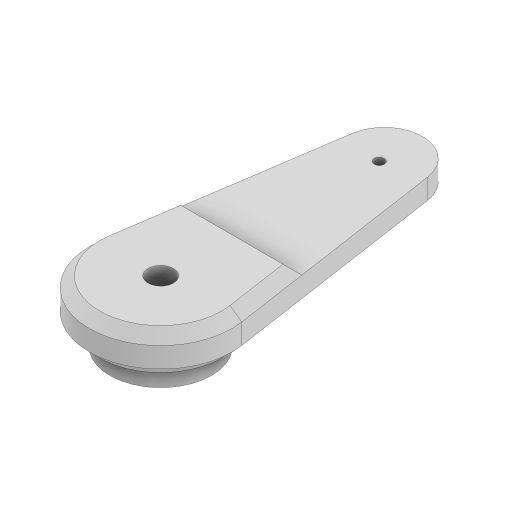
# Autodesk Inventor part: 5P.00.18.01-IB-VTP-Servo-Horn
Saved by Autodesk Inventor 2024.3 (Build 283343000, 343)
## iProperties
Created: 2025-01-15
Part Number: 5P.00.18.01-IB-VTP-Servo-Horn
Material: Generic
Document SubType Name: Modeling
Designer: inigo
Density: 1 g/cm^3
Appearance: Default
Author: inigo
Autodesk Inventor part; units mm, degrees
ref_plane "YZ Plane" through (0, 0, 0) normal (1, 0, 0) x (0, 1, 0)
ref_plane "XZ Plane" through (0, 0, 0) normal (0, 1, 0) x (-1, 0, 0)
sketch "Sketch1" plane through (0, 0, 0) normal (0, 1, 0) x (-1, 0, 0)
  arc A0 (6.9232, -1.0341) -> (-6.9232, -1.0341) centre (0, 0) ccw
  arc A1 (-3.7089, -22.554) -> (3.7089, -22.554) centre (0, -22) ccw
  line L0 (6.9232, -1.0341) -> (3.7089, -22.554)
  line L1 (-6.9232, -1.0341) -> (-3.7089, -22.554)
  circle A2 centre (0, -21.5) radius 0.5
  dimension "d0" = 14
  dimension "d1" = 7.5
  dimension "d2" = 22
  dimension "d3" = 1
  dimension "d4" = 21.5
  constraints: 4 end point, 4 point on circle, 4 tangent, 3 centre point, 2 vertical alignment, 1 coincident
  measures "d0" diameter of A0
  measures "d1" diameter of A1
  measures "d2" distance of A1.centre point (0, 0)
  measures "d3" diameter of A2
  measures "d4" distance of point (0, 0) A2.centre
extrude "Extrusion1" add sketch "Sketch1" along normal blind 2
sketch "Sketch2" plane through (0, 2, 0) normal (0, 1, 0) x (1, 0, 0)
  line L0 (-3.7089, 22.554) -> (-6.9232, 1.0341) projected
  line L1 (-5.8827, 8) -> (5.8827, 8)
  line L2 (6.9232, 1.0341) -> (3.7089, 22.554) projected
  arc A0 (-6.9232, 1.0341) -> (6.9232, 1.0341) centre (0, 0) ccw projected
  dimension "d7" = 8
  constraints: 2 end point, 2 point on line, 1 horizontal
  measures "d7" distance from line of point (0, 0) L1
extrude "Extrusion2" add sketch "Sketch2" along normal blind 1
chamfer "Chamfer1" distance 1 angle 45 3 edges at (6.403, 3, -4.517) (0, 3, 7) (-6.403, 3, -4.517)
chamfer "Chamfer2" distance 1 angle 45 1 edges at (0, 3, -8)
ref_plane "Work Plane1" through (0, 1, 0) normal (0, -1, 0) x (1, 0, 0)
mirror "Mirror1" about plane through (0, 1, 0) normal (0, -1, 0)
sketch "Sketch3" plane through (0, -1, 0) normal (0, -1, 0) x (1, 0, 0)
  circle A0 centre (0, 0) radius 5
  circle A1 centre (0, 0) radius 2.5
  dimension "d17" = 10
  dimension "d18" = 5
  constraints: 2 centre point, 2 coincident
  measures "d17" diameter of A0
  measures "d18" diameter of A1
extrude "Extrusion3" add sketch "Sketch3" along normal blind 2
sketch "Sketch4" plane through (0, 3, 0) normal (0, 1, 0) x (1, 0, 0)
  point P0 (0, 0)
  point P1 (0, 0)
  constraints: 1 coincident
hole "Hole1" at (0, 3, 0) direction (0, -1, 0) diameter 2.5 depth 6
body "Solid1"
